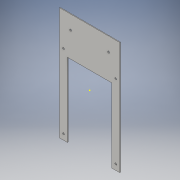
# Autodesk Inventor part: Part2
Saved by Autodesk Inventor 2016 (Build 200138000, 138)
## iProperties
Created: 2015-10-15
Part Number: Part2
Material: Generic
Document SubType Name: Modeling
Designer: hozhu
Density: 1 g/cm^3
Appearance: Default
Author: hozhu
Autodesk Inventor part; units mm, degrees
ref_plane "YZ Plane" through (0, 0, 0) normal (1, 0, 0) x (0, 1, 0)
ref_plane "XZ Plane" through (0, 0, 0) normal (0, 1, 0) x (-1, 0, 0)
ref_plane "XY Plane" through (0, 0, 0) normal (0, 0, 1) x (1, 0, 0)
sketch "Sketch1" plane through (0, 0, 0) normal (0, 0, 1) x (1, 0, 0)
  line L0 (-68.58, -128.7145) -> (68.58, -128.7145)
  line L1 (68.58, -128.7145) -> (68.58, 128.7145)
  line L2 (68.58, 128.7145) -> (-68.58, 128.7145)
  line L3 (-68.58, 128.7145) -> (-68.58, -128.7145)
  line L4 (-68.58, -128.7145) -> (68.58, 128.7145) construction
  line L5 (68.58, -128.7145) -> (-68.58, 128.7145) construction
  point P0 (0, 0)
  dimension "d0" = 137.16
  dimension "d1" = 257.429
  constraints: 12 end point, 2 midpoint, 2 parallel, 1 horizontal, 1 perpendicular
  measures "d0" distance of L1.end L2.end
  measures "d1" distance of L2.end L0.start
extrude "Extrusion1" add sketch "Sketch1" against normal blind 1.5875
sketch "Sketch2" plane through (0, 0, 0) normal (0, 0, 1) x (1, 0, 0)
  circle A0 centre (-59.69, 52.5145) radius 2.0955
  line L0 (-68.58, 128.7145) -> (-68.58, -128.7145) projected
  line L1 (-68.58, 128.7145) -> (68.58, 128.7145) projected
  circle A1 centre (59.69, 52.5145) radius 2.0955
  line L2 (68.58, -128.7145) -> (68.58, 128.7145) projected
  circle A2 centre (-59.69, -116.0145) radius 2.0955
  circle A3 centre (59.69, -116.0145) radius 2.0955
  line L3 (-68.58, -128.7145) -> (68.58, -128.7145) projected
  point P0 (0, 0)
  dimension "d4" = 8.89
  dimension "d5" = 76.2
  dimension "d6" = 76.2
  dimension "d7" = 8.89
  dimension "d8" = 4.191
  dimension "d9" = 12.7
  dimension "d10" = 8.89
  dimension "d11" = 8.89
  dimension "d12" = 12.7
  dimension "d13" = 4.191
  dimension "d21" = 4.191
  dimension "d22" = 4.191
  constraints: 4 centre point
  measures "d4" distance from line of L0 A0.centre
  measures "d5" distance from line of L1 A0.centre
  measures "d6" distance from line of L1 A1.centre
  measures "d7" distance from line of A1.centre L2
  measures "d8" diameter of A1
  measures "d9" distance from line of L3 A2.centre
  measures "d10" distance from line of L0 A2.centre
  measures "d11" distance from line of L2 A3.centre
  measures "d12" distance from line of L3 A3.centre
  measures "d13" diameter of A0
  measures "d21" diameter of A2
  measures "d22" diameter of A3
hole "Hole1" at (-59.69, 52.5145, 0) at (59.69, 52.5145, 0) at (-59.69, -116.0145, 0) at (59.69, -116.0145, 0) direction (0, 0, -1) diameter 4.191 end through all
sketch "Sketch4" plane through (0, 0, 0) normal (0, 0, 1) x (1, 0, 0)
  line L0 (-35.179, -49.0855) -> (-35.179, -99.8855)
  line L1 (-28.321, -49.0855) -> (-28.321, -99.8855)
  line L2 (28.321, -49.0855) -> (28.321, -99.8855)
  line L3 (35.179, -49.0855) -> (35.179, -99.8855)
  line L4 (-68.58, 128.7145) -> (-68.58, -128.7145) projected
  line L5 (68.58, -128.7145) -> (68.58, 128.7145) projected
  line L6 (-68.58, -128.7145) -> (68.58, -128.7145) projected
  arc A0 (-28.321, -49.0855) -> (-35.179, -49.0855) centre (-31.75, -49.0855) ccw
  arc A1 (-35.179, -99.8855) -> (-28.321, -99.8855) centre (-31.75, -99.8855) ccw
  arc A2 (35.179, -49.0855) -> (28.321, -49.0855) centre (31.75, -49.0855) ccw
  arc A3 (28.321, -99.8855) -> (35.179, -99.8855) centre (31.75, -99.8855) ccw
  point P0 (0, 0)
  dimension "d23" = 6.858
  dimension "d24" = 6.858
  dimension "d25" = 33.401
  dimension "d26" = 50.8
  dimension "d27" = 33.401
  dimension "d28" = 28.829
  dimension "d29" = 28.829
  dimension "d30" = 28.829
  dimension "d31" = 28.829
  dimension "d32" = 50.8
  dimension "d33" = 50.8
  dimension "d34" = 50.8
  constraints: 8 end point, 8 point on circle, 4 centre point, 4 tangent, 4 vertical
  measures "d23" distance of L1.end L0.end
  measures "d24" distance between parallel lines of L3 L2
  measures "d25" distance between parallel lines of L4 L0
  measures "d26" distance of L3.start L3.end
  measures "d27" distance between parallel lines of L5 L3
  measures "d28" distance from line of L6 L0.end
  measures "d29" distance from line of L6 L1.end
  measures "d30" distance from line of L6 L2.end
  measures "d31" distance from line of L6 L3.end
  measures "d32" distance of L0.start L0.end
  measures "d33" distance of L1.start L1.end
  measures "d34" distance of L2.start L2.end
extrude "Extrusion2" cut sketch "Sketch4" against normal blind 3.175
sketch "Sketch5" plane through (0, 0, 0) normal (0, 0, 1) x (1, 0, 0)
  line L0 (-68.58, 128.7145) -> (68.58, 128.7145) projected
  line L1 (68.58, 128.7145) -> (68.58, -128.7145) projected
  point P0 (0, 0)
  point P1 (-43.3324, 96.9645)
  point P2 (43.3324, 96.9645)
  dimension "d37" = 31.75
  dimension "d38" = 86.6648
  dimension "d39" = 31.75
  dimension "d40" = 25.2476
  measures "d37" distance from line of L0 point (-43.332, 96.964)
  measures "d38" distance of point (-43.332, 96.964) point (43.332, 96.964)
  measures "d39" distance from line of L0 point (43.332, 96.964)
  measures "d40" distance from line of L1 point (43.332, 96.964)
hole "Hole2" at (-43.3324, 96.9645, 0) at (43.3324, 96.9645, 0) direction (0, 0, -1) diameter 4.4704 end through all
sketch "battery_buzzer" plane through (0, 0, 0) normal (0, 0, 1) x (1, 0, 0)
  point P0 (0, 0)
sketch "Sketch10" plane through (0, 0, 0) normal (0, 0, 1) x (1, 0, 0)
  line L0 (-50.8, -128.7145) -> (-50.8, 39.8145)
  line L1 (-50.8, 39.8145) -> (50.8, 39.8145)
  line L2 (50.8, 39.8145) -> (50.8, -128.7145)
  line L3 (68.58, 128.7145) -> (-68.58, 128.7145) projected
  line L4 (-68.58, 128.7145) -> (-68.58, -128.7145) projected
  line L5 (68.58, 128.7145) -> (68.58, -128.7145) projected
  line L6 (-50.8, -128.7145) -> (50.8, -128.7145)
  point P0 (0, 0)
  dimension "d48" = 88.9
  dimension "d49" = 17.78
  dimension "d50" = 17.78
  constraints: 8 end point, 3 perpendicular, 1 vertical
  measures "d48" distance between parallel lines of L3 L1
  measures "d49" distance between parallel lines of L4 L0
  measures "d50" distance between parallel lines of L5 L2
extrude "Extrusion3" cut sketch "Sketch10" against normal blind 3.175
body "Solid1"
